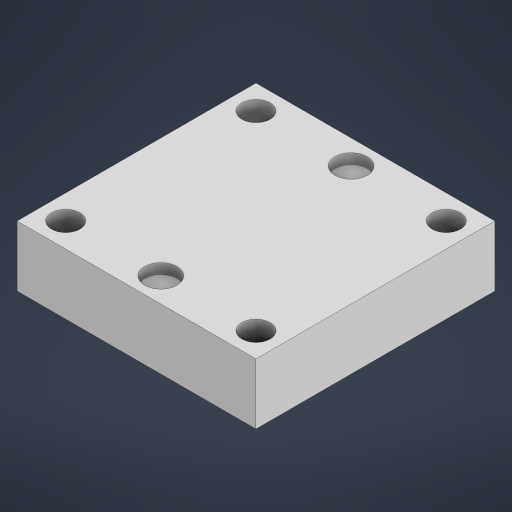
# Autodesk Inventor part: antennaTripodMount
Saved by Autodesk Inventor 2024 (Build 280153000, 153)
## iProperties
Created: 2024-02-10
Part Number: antennaTripodMount
Material: Generic
Document SubType Name: Modeling
Designer: madis
Density: 1 g/cm^3
Appearance: Default
Author: madis
Autodesk Inventor part; units mm, degrees
ref_plane "YZ Plane" through (0, 0, 0) normal (1, 0, 0) x (0, 1, 0)
ref_plane "XZ Plane" through (0, 0, 0) normal (0, 1, 0) x (-1, 0, 0)
ref_plane "XY Plane" through (0, 0, 0) normal (0, 0, 1) x (1, 0, 0)
sketch "Sketch1" plane through (0, 0, 0) normal (0, 1, 0) x (-1, 0, 0)
  line L0 (37.5, 37.5) -> (-37.5, 37.5)
  line L1 (-37.5, 37.5) -> (-37.5, -37.5)
  line L2 (-37.5, -37.5) -> (37.5, -37.5)
  line L3 (37.5, -37.5) -> (37.5, 37.5)
  point P0 (0, 0)
  dimension "d0" = 75
  dimension "d1" = 75
  dimension "d2" = 37.5
  dimension "d3" = 37.5
  constraints: 8 end point, 2 parallel, 1 horizontal, 1 perpendicular
  measures "d0" distance of L2.end L0.start
  measures "d1" distance of L0.start L0.end
  measures "d2" distance from line of point (0, 0) L3
  measures "d3" distance from line of point (0, 0) L0
extrude "Extrusion1" add sketch "Sketch1" along normal blind 19.05
sketch "Sketch3" plane through (0, 19.05, 0) normal (0, 1, 0) x (1, 0, 0)
  line L0 (-37.5, 37.5) -> (-37.5, -37.5) projected
  line L1 (37.5, 37.5) -> (-37.5, 37.5) projected
  point P0 (0, 0)
  point P1 (-29.88, 29.88)
  dimension "d27" = 7.62
  dimension "d28" = 7.62
  measures "d27" distance from line of L0 point (-29.88, 29.88)
  measures "d28" distance from line of L1 point (-29.88, 29.88)
hole "Hole2" at (-29.88, 19.05, -29.88) direction (0, -1, 0) diameter 8.89 depth 11.43
pattern_linear "Rectangular Pattern1" count 2 spacing 59.76 along (1, 0, 0) count 2 spacing 59.76 along (0, 0, 1) of "Hole2"
sketch "Sketch4" plane through (0, 19.05, 0) normal (0, 1, 0) x (1, 0, 0)
  line L0 (37.5, 37.5) -> (-37.5, 37.5) projected
  point P0 (0, 0)
  point P1 (0, 29.88)
  dimension "d36" = 0
  dimension "d37" = 7.62
  measures "d36" horizontal distance of point (0, 0) point (0, 29.88)
  measures "d37" distance from line of L0 point (0, 29.88)
hole "Hole3" at (0, 19.05, -29.88) direction (0, -1, 0) diameter 10.16 depth 3.175
mirror "Mirror1" about plane through (0, 0, 0) normal (0, 0, 1) of "Hole3"
sketch "Sketch5" plane through (0, 0, 0) normal (0, -1, 0) x (1, 0, 0)
  point P0 (0, 0)
  point P1 (0, 0)
  constraints: 1 coincident
hole "Hole4" at (0, 0, 0) direction (0, 1, 0) diameter 8.89 depth 11.43
body "Solid1"
